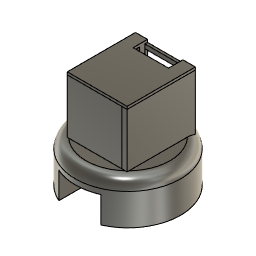
surface temperature sensor (Autodesk Fusion 360 design; units mm, degrees)
Autodesk Fusion 360 part; units mm, degrees
sketch "Sketch1" plane through (0, 0, 0) normal (0, 0, 1) x (1, 0, 0)
  circle A0 centre (0, 0) radius 20
  circle A1 centre (0, 0) radius 3.5
  line L0 (0, 0) -> (0, 6) construction
  line L1 (0, 6) -> (3, 6) construction
  circle A2 centre (3, 6) radius 1.4
  circle A3 centre (-3, 6) radius 1.4
  circle A4 centre (3, 6) radius 1.9
  circle A5 centre (-3, 6) radius 1.9
  line L2 (3, 6) -> (3, -9.2119) construction
  circle A6 centre (0, 0) radius 4.5 construction
  circle A7 centre (3.5116, -4.7509) radius 1
  circle A8 centre (-3.5116, -4.7509) radius 1
  line L3 (0, 0) -> (8, 0) construction
  line L4 (0, 0) -> (0, 12.8) construction
  line L5 (8, 12.6629) -> (8, -10.3371)
  line L6 (8, 12.6629) -> (-9.8, 12.6629)
  line L7 (-9.8, 12.6629) -> (-9.8, -10.3371)
  line L8 (-9.8, -10.3371) -> (8, -10.3371)
  line L9 (-9.8, 8.6629) -> (8, 8.6629) construction
  line L10 (-11.3, 14.1629) -> (-11.3, -11.8371)
  line L11 (-11.3, -11.8371) -> (9.5, -11.8371)
  line L12 (9.5, 14.1629) -> (9.5, -11.8371)
  line L13 (9.5, 14.1629) -> (-11.3, 14.1629)
  line L14 (-10.3, -10.8371) -> (8.5, -10.8371)
  line L15 (8.5, 13.1629) -> (8.5, -10.8371)
  line L16 (8.5, 13.1629) -> (-10.3, 13.1629)
  line L17 (-10.3, 13.1629) -> (-10.3, -10.8371)
  dimension "d1" = 40
  dimension "d2" = 7
  dimension "d3" = 6
  dimension "d4" = 3
  dimension "d5" = 2.8
  dimension "d10" = 0.5
  dimension "d11" = 0.5
  dimension "d14" = 9
  dimension "d15" = 2
  dimension "d24" = 8
  dimension "d25" = 12.8
  dimension "d26" = 17.8
  dimension "d27" = 23
  dimension "d28" = 4
  dimension "d31" = 1.5
  dimension "d32" = 0.5
  constraint coincident A0.centre A1.centre
  constraint concentric A0 A1
  constraint vertical L0
  constraint perpendicular L0 L1
  constraint coincident L1.end A2.centre
  constraint symmetric L0 A2 A3
  constraint symmetric L0 A7 A8
  constraint horizontal L3
  constraint perpendicular L5 L6
  constraint perpendicular L6 L7
  constraint horizontal L9
  constraint coincident L5 L9.end
  measures "d1" diameter of A0
  measures "d2" diameter of A1
  measures "d3" distance of A0.centre L0.end
  measures "d4" distance of L0.end L1.end
  measures "d5" diameter of A2
  measures "d14" diameter of A6
  measures "d15" diameter of A7
  measures "d24" distance of A0.centre L3.end
  measures "d25" distance of A0.centre L4.end
  measures "d26" distance of L5.start L6.end
  measures "d27" distance of L6.end L7.end
  measures "d28" distance of L6.end L9.start
extrude "Extrude1" add sketch "Sketch1" against normal blind 1 contours A0 | A4 | A5 | A7 | A8 | L5 L6 L7 L8 | L10 L11 L12 L13 | L14 L15 L16 L17 makes body 1
extrude "Extrude2" add sketch "Sketch1" 1 faces at (-9.1663, 2.965, 0) against normal blind 1 contours A2 | A3 on bodies 1 bodies 1
extrude "Extrude3" add sketch "Sketch1" along normal blind 5 contours A2 | A3 | A4 | A5 bodies 1
extrude "Extrude4" add sketch "Sketch1" along normal blind 5 contours A7 | A8 bodies 1
extrude "Extrude5" add sketch "Sketch1" along normal blind 8 separate body contours A2 | A3 makes body 2 at (-1.6017, 5.9302, 5.3333) makes body 3 at (4.3983, 5.9302, 5.3333)
combine "Combine1" operation add target body 2 tool bodies 1 3
sketch "Sketch2" plane through (0, 0, -1) normal (0, 0, -1) x (1, 0, 0)
  circle A0 centre (0, 0) radius 3.5
  circle A1 centre (0, 0) radius 20
  line L0 (-20, -0.0143) -> (-8, -0.0143) construction
  line L1 (20, 0.0006) -> (8, 0.0006) construction
  line L2 (-8, 18.3303) -> (-8, -18.3303)
  line L3 (8, 18.3303) -> (8, -18.3303)
  dimension "d20" = 12
  dimension "d21" = 12
  constraint coincident A1 L0.start
  constraint horizontal L0
  constraint coincident A1 L1.start
  constraint horizontal L1
  constraint coincident A1 L2.start
  constraint coincident A1 L2.end
  constraint perpendicular L0 L2
  constraint coincident A1 L3.start
  constraint coincident A1 L3.end
  constraint perpendicular L1 L3
  measures "d20" distance of L0.start L0.end
  measures "d21" distance of L1.start L1.end
extrude "Extrude6" add sketch "Sketch2" along normal blind 10 contours A1 L3 | A1 L2 bodies 2
extrude "Extrude7" add sketch "Sketch1" along normal blind 5 separate body contours A0 makes body 4
extrude "Extrude8" add sketch "Sketch1" along normal blind 25 contours L10 L11 L12 L13 bodies 2 4
extrude "Extrude9" add 1 faces at (9.1667, -2.8371, 25) along direction (0, 0, 1) blind 0.1 on bodies 2 bodies 2
sketch "Sketch3" plane through (0, -11.8371, 0) normal (0, -1, 0) x (1, 0, 0)
  line L0 (-11.3, 5) -> (9.5, 5)
  line L1 (9.5, 5) -> (9.5, 25.1)
  line L2 (9.5, 25.1) -> (-11.3, 25.1)
  line L3 (-11.3, 25.1) -> (-11.3, 5)
sketch "Sketch4" plane through (0, 14.1629, 0) normal (0, 1, 0) x (-1, 0, 0)
  line L0 (-9.5, 5) -> (11.3, 5)
  line L1 (11.3, 5) -> (11.3, 25.1)
  line L2 (11.3, 25.1) -> (-9.5, 25.1)
  line L3 (-9.5, 25.1) -> (-9.5, 5)
extrude "Extrude10" add 1 faces at (9.5, 5.4963, 11.7) along direction (1, 0, 0) blind 2 on bodies 2 bodies 2
fillet "Fillet1" radius 4 1 edges at (-18.6465, -7.2323, 5) on bodies 2 4
sketch "Sketch5" plane through (0, 14.1629, 0) normal (0, 1, 0) x (-1, 0, 0)
  line L0 (-7.4563, 24) -> (7.3916, 24)
  line L1 (7.3916, 24) -> (7.3916, 7.7953)
  line L2 (7.3916, 7.7953) -> (-7.4563, 7.7953)
  line L3 (-7.4563, 7.7953) -> (-7.4563, 24)
  constraint horizontal L0
  constraint vertical L1
  constraint horizontal L2
  constraint vertical L3
extrude "Extrude11" cut sketch "Sketch5" against normal blind 1 bodies 2
extrude "Extrude12" add 1 faces at (2.5106, 6.5047, 8) along direction (0, 0, 1) blind 2 on bodies 2 bodies 2
extrude "Extrude13" add 1 faces at (10.5, -2.8371, 25.1) along direction (0, 0, 1) blind 0.5 on bodies 2 bodies 2
extrude "Extrude14" add 1 faces at (-2.4423, 13.4963, 7.7953) along direction (0, 0, 1) blind 3 on bodies 2 bodies 2
extrude "Extrude15" add 1 faces at (7.4563, 13.8296, 15.1968) along direction (-1, 0, 0) blind 0.7 on bodies 2 bodies 2
extrude "Extrude16" add 1 faces at (-7.3916, 13.8296, 19.5984) along direction (1, 0, 0) blind 0.7 on bodies 2 bodies 2
extrude "Extrude17" add sketch "Sketch1" along normal blind 25.5 contours L14 L15 L16 L17 bodies 2
extrude "Extrude18" add 1 faces at (-3.8667, -10.3371, 8.5) along direction (0, -1, 0) blind 1 on bodies 2 bodies 2
extrude "Extrude19" add 1 faces at (-3.8667, -10.3371, 8.5) along direction (0, -1, 0) blind 1 on bodies 2 bodies 2
extrude "Extrude20" add 1 faces at (8.3333, -2.6704, 25.5) along direction (0, 0, 1) blind 0.1 on bodies 2 bodies 2
extrude "Extrude21" cut 1 faces at (-2.209, 13.1629, 19.5984) along direction (0, -1, 0) blind 2 on bodies 2 bodies 2
ref_plane "WorkPlane1" through (0.1, 1.1629, 39.6) normal (0, 0, 1) x (1, 0, 0)
sketch "Sketch6" plane through (0.1, 1.1629, 39.6) normal (0, 0, 1) x (1, 0, 0)
  line L0 (-11.4, 13, -14) -> (11.4, 13, -14)
  line L1 (11.4, 13, -14) -> (11.4, -13, -14)
  line L2 (11.4, -13, -14) -> (-11.4, -13, -14)
  line L3 (-11.4, -13, -14) -> (-11.4, 13, -14)
  line L4 (-9.9, 11.5, -14) -> (7.9, 11.5, -14)
  line L5 (7.9, 11.5, -14) -> (7.9, -11.5, -14)
  line L6 (7.9, -11.5, -14) -> (-9.9, -11.5, -14)
  line L7 (-9.9, -11.5, -14) -> (-9.9, 11.5, -14)
ref_plane "WorkPlane2" through (0.1, 1.1629, 58.6) normal (0, 0, 1) x (1, 0, 0)
sketch "Sketch7" plane through (0.1, 1.1629, 58.6) normal (0, 0, 1) x (1, 0, 0)
  line L0 (7.9, 11.5) -> (7.9, -11.5)
  line L1 (11.4, 13) -> (11.4, -13)
  line L2 (11.4, -13) -> (-11.4, -13)
  line L3 (-9.9, -11.5) -> (-9.9, 11.5)
  line L4 (-11.4, -13) -> (-11.4, 13)
  line L5 (7.9, -11.5) -> (-9.9, -11.5)
  line L6 (-9.9, 11.5) -> (7.9, 11.5)
  line L7 (-11.4, 13) -> (11.4, 13)
  line L8 (-8.4, 10) -> (6.4, 10)
  line L9 (6.4, 10) -> (6.4, -10)
  line L10 (6.4, -10) -> (-8.4, -10)
  line L11 (-8.4, -10) -> (-8.4, 10)
  dimension "d67" = 1.5
extrude "Extrude22" add sketch "Sketch7" along normal blind 1 separate body contours L0 L3 L5 L6 | L1 L2 L4 L7 | L8 L9 L10 L11 makes body 5
extrude "Extrude23" add sketch "Sketch7" against normal blind 2 contours L0 L3 L5 L6 bodies 5
extrude "Extrude24" cut sketch "Sketch1" along normal blind 27 contours L14 L15 L16 L17 bodies 2
sketch "Sketch8" plane through (0, 0, 10) normal (0, 0, 1) x (-1, 0, 0)
  circle A0 centre (-3, -6) radius 1.4
  line L0 (10.3, -13.16) -> (-8.5, -13.16)
  line L1 (-8.5, -13.16) -> (-8.5, 10.8375)
  line L2 (-8.5, 10.8375) -> (10.3, 10.8375)
  line L3 (10.3, 10.8375) -> (10.3, -13.16)
  constraint horizontal L0
  constraint vertical L1
  constraint horizontal L2
  constraint vertical L3
sketch "Sketch9" plane through (0, 0, 59.6) normal (0, 0, 1) x (-1, 0, 0)
  line L0 (11.3, -14.1629) -> (11.3, 11.8371)
  line L1 (11.3, 11.8371) -> (-11.5, 11.8371)
  line L2 (-11.5, 11.8371) -> (-11.5, -14.1629)
  line L3 (-11.5, -14.1629) -> (11.3, -14.1629)
  line L4 (10.3, -13.15) -> (-8.5, -13.15)
  line L5 (-8.5, -13.15) -> (-8.5, 10.8)
  line L6 (-8.5, 10.8) -> (10.3, 10.8)
  line L7 (10.3, 10.8) -> (10.3, -13.15)
  constraint horizontal L4
  constraint vertical L5
  constraint horizontal L6
  constraint vertical L7
extrude "Extrude25" add sketch "Sketch9" against normal blind 3 contours L4 L5 L6 L7 bodies 5
extrude "Extrude26" cut sketch "Sketch7" against normal blind 3 contours L8 L9 L10 L11 bodies 5
move_body "Move1" bodies 5 to x (1, 0, 0) y (0, 1, 0) z (0, 0, 1) at (0, 0, -18)
extrude "Extrude27" cut 1 faces at (6.5, 4.4963, 39.9333) along direction (1, 0, 0) blind 0.5 on bodies 5 bodies 5
extrude "Extrude28" cut 1 faces at (-8.3, -2.1704, 39.9333) along direction (-1, 0, 0) blind 0.5 on bodies 5 bodies 5
move_body "Move2" bodies 5 to x (1, 0, 0) y (0, 1, 0) z (0, 0, 1) at (0, 0, 22)
move_body "Move3" bodies 5 to x (1, 0, 0) y (0, 1, 0) z (0, 0, 1) at (0, 0, 85)
sketch "Sketch10" plane through (0, 0, 148.6) normal (0, 0, 1) x (-1, 0, 0)
  line L0 (11.3, -14.1629) -> (11.3, 11.8371)
  line L1 (11.3, 11.8371) -> (-11.5, 11.8371)
  line L2 (-11.5, 11.8371) -> (-11.5, -14.1629)
  line L3 (-11.5, -14.1629) -> (11.3, -14.1629)
  line L4 (6.7164, -14.1629) -> (-6.7549, -14.1629)
  line L5 (-6.7549, -14.1629) -> (-6.7549, -8.6629)
  line L6 (-6.7549, -8.6629) -> (6.7164, -8.6629)
  line L7 (6.7164, -8.6629) -> (6.7164, -14.1629)
  dimension "d82" = 5.5
  constraint horizontal L4
  constraint vertical L5
  constraint horizontal L6
  constraint vertical L7
  constraint coincident L3 L4.start
  measures "d82" distance of L4.start L6.end
extrude "Extrude29" cut sketch "Sketch10" against normal blind 3 contours L3 L4 L5 L6 L7 bodies 5
extrude "Extrude30" cut 1 faces at (2.5106, 6.5047, 10) along direction (0, 0, -1) blind 1 on bodies 2 bodies 2
extrude "Extrude31" cut 1 faces at (2.5106, 6.5047, 9) along direction (0, 0, -1) blind 0.5 on bodies 2 bodies 2
extrude "Extrude32" add 1 faces at (-3.5333, -10.1457, 145.6) along direction (0, 0, -1) blind 1 on bodies 5 bodies 5
move_body "Move4" bodies 5 to x (1, 0, 0) y (0, 1, 0) z (0, 0, 1) at (0, 0, -120)
move_body "Move5" bodies 5 to x (1, 0, 0) y (0, 1, 0) z (0, 0, 1) at (0, 0, -2)
